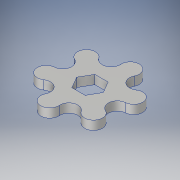
# Autodesk Inventor part: Turret Drive Gear
Saved by Autodesk Inventor 2019.4 (Build 234330000, 330)
## iProperties
Created: 2020-01-29
Part Number: Turret Drive Gear
Material: Aluminum 6061
Document SubType Name: Modeling
Designer: admin
Density: 2.7 g/cm^3
Appearance: Aluminum - Flat
Author: admin
Autodesk Inventor part; units mm, degrees
ref_plane "YZ Plane" through (0, 0, 0) normal (1, 0, 0) x (0, 1, 0)
ref_plane "XZ Plane" through (0, 0, 0) normal (0, 1, 0) x (-1, 0, 0)
ref_plane "XY Plane" through (0, 0, 0) normal (0, 0, 1) x (1, 0, 0)
sketch "Sketch1" plane through (0, 0, 0) normal (0, 1, 0) x (-1, 0, 0)
  circle A0 centre (0, 0) radius 19.3185 construction
  arc A1 (18.6108, 1.3574) -> (20.8827, 10.5931) centre (18.2471, 6.3441) ccw
  arc A2 (18.6108, 1.3574) -> (16.7961, -8.1299) centre (18.9745, -3.6294) ccw
  arc A3 (10.4809, -15.4388) -> (16.7961, -8.1299) centre (14.6177, -12.6304) ccw
  arc A4 (10.4809, -15.4388) -> (1.3574, -18.6108) centre (6.3441, -18.2471) ccw
  arc A5 (-4.0919, -23.9531) -> (1.3574, -18.6108) centre (-3.6294, -18.9745) ccw
  line L0 (14.0636, -2.69) -> (0, 0)
  line L1 (0, 0) -> (4.7021, -13.5244)
  dimension "d0" = 5
  dimension "d1" = 5
  dimension "d2" = 5
  dimension "d3" = 5
  dimension "d4" = 5
  dimension "d5" = 60
  constraints: 17 point on circle, 6 centre point, 4 end point, 4 equal radius, 1 coincident
  measures "d0" radius of A1
  measures "d1" radius of A2
  measures "d2" radius of A3
  measures "d3" radius of A4
  measures "d4" radius of A5
  measures "d5" angle of L1 L0
extrude "Extrusion1" add sketch "Sketch1" along normal blind 5
pattern_circular "Circular Pattern1" count 6 over 360 about axis through (0, 0, 0) along (0, 1, 0) of "Extrusion1"
sketch "Sketch2" plane through (0, 5, 0) normal (0, 1, 0) x (1, 0, 0)
  line L0 (3.7239, 6.45) -> (7.4478, 0)
  line L1 (7.4478, 0) -> (3.7239, -6.45)
  line L2 (3.7239, -6.45) -> (-3.7239, -6.45)
  line L3 (-3.7239, -6.45) -> (-7.4478, 0)
  line L4 (-7.4478, 0) -> (-3.7239, 6.45)
  line L5 (-3.7239, 6.45) -> (3.7239, 6.45)
  point P0 (0, 0)
  point P1 (0, 0)
  dimension "d11" = 12.9
  constraints: 12 end point, 1 coincident, 1 horizontal, 13 other
  measures "d11" distance between parallel lines of L4 L1
extrude "Extrusion2" cut sketch "Sketch2" against normal up to surface (5 mm away)
equation "\"d1\" = d0"
equation "\"d2\" = d0"
equation "\"d3\" = d0"
equation "\"d4\" = d0"
body "Solid1"
